lacznik podstawa pokrywa krutki v2 (Autodesk Fusion 360 design; units mm, degrees)
Autodesk Fusion 360 part; units mm, degrees
sketch "Sketch1" plane through (0, 0, 0) normal (0, 0, 1) x (1, 0, 0) in component "czniki podstawy z pokryw"
  line L0 (0, 0) -> (41.5, 0)
  line L1 (41.5, 0) -> (41.5, 6)
  line L2 (41.5, 6) -> (0, 6)
  line L3 (0, 6) -> (0, 0)
  line L4 (0, 3) -> (41.5, 3) construction
  circle A0 centre (4, 3) radius 2
  circle A1 centre (37.5, 3) radius 2
  dimension "d1" = 4
  dimension "d2" = 4
  dimension "d3" = 33.5
  dimension "d4" = 4
  dimension "d5" = 4
  dimension "d6" = 3
  constraint horizontal L0
  constraint vertical L1
  constraint horizontal L2
  constraint vertical L3
  constraint coincident L0.start L3.end
  constraint midpoint L3 L4.start
  constraint midpoint L1 L4.end
  constraint coincident L4 A0.centre
  constraint coincident L4 A1.centre
  measures "d1" diameter of A0
  measures "d2" diameter of A1
  measures "d3" distance of A0.centre A1.centre
  measures "d4" distance of L3 A0.centre
  measures "d5" distance of L1 A1.centre
  measures "d6" distance of L2 A0.centre
extrude "Extrude1" add sketch "Sketch1" along normal blind 8 makes body 1 in component "czniki podstawy z pokryw"
sketch "Sketch2" plane through (0, 0, 0) normal (0, -1, 0) x (1, 0, 0) in component "czniki podstawy z pokryw"
  line L0 (0, 0) -> (41.5, 0)
  line L1 (41.5, 0) -> (41.5, 8)
  line L2 (41.5, 8) -> (0, 8)
  line L3 (0, 8) -> (0, 0)
  line L4 (20.75, 0) -> (20.75, 8) construction
  circle A0 centre (20.75, 5) radius 2
  dimension "d9" = 4
  dimension "d10" = 5
  constraint midpoint L2 L4.end
  constraint midpoint L0 L4.start
  constraint coincident L4 A0.centre
  measures "d9" diameter of A0
  measures "d10" distance of L0 A0.centre
extrude "Extrude2" cut sketch "Sketch2" against normal blind 6 contours A0 bodies 1 in component "czniki podstawy z pokryw"
sketch "Sketch1 (2)" plane through (0, 0, 0) normal (0, 0, 1) x (1, 0, 0) in component "czniki podstawy z pokryw dlurzszy"
  line L0 (0, 0) -> (41.5, 0)
  line L1 (41.5, 0) -> (41.5, 6)
  line L2 (41.5, 6) -> (0, 6)
  line L3 (0, 6) -> (0, 0)
  line L4 (0, 3) -> (41.5, 3) construction
  circle A0 centre (4, 3) radius 2
  circle A1 centre (37.5, 3) radius 2
  dimension "d1_1" = 4
  dimension "d2_1" = 4
  dimension "d3_1" = 33.5
  dimension "d4_1" = 4
  dimension "d5_1" = 4
  dimension "d6_1" = 3
  constraint horizontal L0
  constraint vertical L1
  constraint horizontal L2
  constraint vertical L3
  constraint coincident L0.start L3.end
  constraint midpoint L3 L4.start
  constraint midpoint L1 L4.end
  constraint coincident L4 A0.centre
  constraint coincident L4 A1.centre
  measures "d1_1" diameter of A0
  measures "d2_1" diameter of A1
  measures "d3_1" distance of A0.centre A1.centre
  measures "d4_1" distance of L3 A0.centre
  measures "d5_1" distance of L1 A1.centre
  measures "d6_1" distance of L2 A0.centre
extrude "Extrude1'" add sketch "Sketch1 (2)" along normal blind 8 separate body makes body 2 in component "czniki podstawy z pokryw dlurzszy"
sketch "Sketch2 (2)" plane through (0, 0, 0) normal (0, -1, 0) x (1, 0, 0) in component "czniki podstawy z pokryw dlurzszy"
  line L0 (0, 0) -> (41.5, 0)
  line L1 (41.5, 0) -> (41.5, 8)
  line L2 (41.5, 8) -> (0, 8)
  line L3 (0, 8) -> (0, 0)
  line L4 (20.75, 0) -> (20.75, 8) construction
  circle A0 centre (20.75, 5) radius 2
  dimension "d9_1" = 4
  dimension "d10_1" = 5
  constraint midpoint L2 L4.end
  constraint midpoint L0 L4.start
  constraint coincident L4 A0.centre
  measures "d9_1" diameter of A0
  measures "d10_1" distance of L0 A0.centre
extrude "Extrude2'" cut sketch "Sketch2 (2)" against normal blind 6 contours A0 bodies 2 in component "czniki podstawy z pokryw dlurzszy"
extrude "Extrude3" add 1 faces at (6.2574, 0, 4.234) along direction (0, -1, 0) blind 2 on bodies 2 bodies 2 in component "czniki podstawy z pokryw dlurzszy"
component "czniki podstawy z pokryw" placed x (1, 0, 0) y (0, 1, 0) z (0, 0, 1) at (0, 0, 0)
component "czniki podstawy z pokryw dlurzszy" placed x (1, 0, 0) y (0, 1, 0) z (0, 0, 1) at (0, 0, -24)
